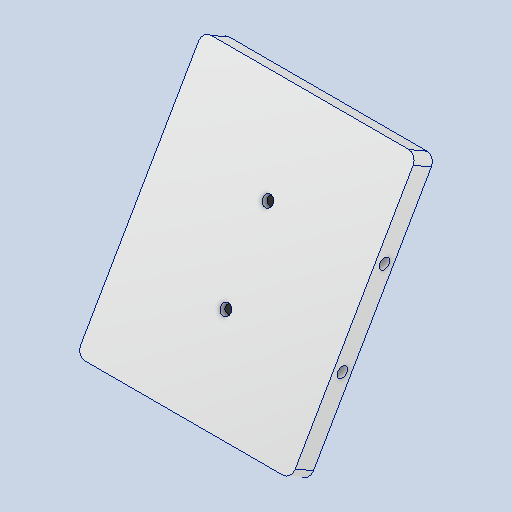
# Autodesk Inventor part: belt_liner_v5_Plate_3
Saved by Autodesk Inventor 2025.2 (Build 292293000, 293)
## iProperties
Created: 2025-02-23
Part Number: belt_liner_v5_Plate_3
Material: アルミニウム 6061
Document SubType Name: Modeling
Designer: haruy
Density: 2.7 g/cm^3
Appearance: アルミニウム - フラット
Author: haruy
Autodesk Inventor part; units mm, degrees
ref_plane "YZ Plane" through (0, 0, 0) normal (1, 0, 0) x (0, 1, 0)
ref_plane "XZ Plane" through (0, 0, 0) normal (0, 1, 0) x (-1, 0, 0)
ref_plane "XY Plane" through (0, 0, 0) normal (0, 0, 1) x (1, 0, 0)
derived "belt_liner_v5_Sketch_Base.ipt"
sketch "スケッチ1" plane through (300, 0, 0) normal (1, 0, 0) x (0, 1, 0)
  circle A0 centre (0, 0) radius 22.36 projected
  circle A1 centre (742.4003, -428.625) radius 23.875 construction
  line L0 (0, 0) -> (0, -985.832) projected
  line L1 (0, 0) -> (742.4003, -428.625) projected
  line L2 (-48.7433, -24.4258) -> (-56.2433, -37.4162) projected
  line L3 (-56.2433, -37.4162) -> (725.7777, -488.9162) projected
  line L4 (725.7777, -488.9162) -> (733.2777, -475.9258) projected
  line L5 (733.2777, -475.9258) -> (-48.7433, -24.4258) projected
  line L6 (-44.1225, 123.2584) -> (-44.1225, 123.2584) projected
  line L7 (0, -985.832) -> (0, 0) projected
  circle A2 centre (0, 0) radius 12.5 projected
  circle A3 centre (0, 0) radius 15 projected
  line L8 (0, 0) -> (0, 0) projected
  circle A4 centre (0, 0) radius 24.06 construction
  line L9 (0, 0) -> (0, 0) projected
  line L10 (0, 0) -> (0, 0) projected
  line L11 (-48.7433, -24.4258) -> (-46.2433, -20.0957) projected
  circle A5 centre (742.4003, -428.625) radius 5 projected
  line L12 (733.2777, -475.9258) -> (707.2969, -460.9258) projected
  line L13 (707.2969, -460.9258) -> (709.7969, -456.5957) projected
  line L14 (709.7969, -456.5957) -> (735.7777, -471.5957) projected
  line L15 (735.7777, -471.5957) -> (733.2777, -475.9258) projected
  circle A6 centre (738.0702, -426.125) radius 5.1 projected
  line L16 (742.4003, -428.625) -> (509.0943, -293.9257) projected
  circle A7 centre (759.7208, -438.625) radius 5.1 projected
  line L17 (740.6202, -421.7083) -> (762.2708, -434.2083) projected
  line L18 (735.5202, -430.5417) -> (757.1708, -443.0417) projected
  circle A8 centre (742.4003, -428.625) radius 22.175 construction
  circle A9 centre (738.0702, -426.125) radius 10.1 construction
  circle A10 centre (759.7208, -438.625) radius 10.1 construction
  line L19 (743.1202, -417.3781) -> (764.7708, -429.8781) construction
  line L20 (733.0202, -434.8719) -> (754.6708, -447.3719) construction
  line L21 (743.1202, -417.3781) -> (730.6598, -410.1842) construction
  line L22 (729.3233, -421.075) -> (734.3733, -412.3281) construction
  line L23 (764.7708, -429.8781) -> (770.9335, -433.4362) construction
  line L24 (770.9335, -433.4362) -> (771.2695, -433.6302) projected
  line L25 (754.6708, -447.3719) -> (764.7708, -429.8781) projected
  line L26 (764.7708, -429.8781) -> (773.431, -434.8781) projected
  line L27 (773.431, -434.8781) -> (763.331, -452.3719) projected
  line L28 (763.331, -452.3719) -> (754.6708, -447.3719) construction
  circle A11 centre (725.8674, -468.7607) radius 1.5 projected
  circle A12 centre (0, 0) radius 30 projected
  circle A13 centre (742.4003, -428.625) radius 6 construction
  circle A14 centre (0, 0) radius 24.06 construction
  circle A15 centre (0, 0) radius 24.06 projected
  circle A16 centre (742.4003, -428.625) radius 24.06 projected
  line L29 (754.4303, -407.7884) -> (12.03, 20.8366) projected
  circle A17 centre (725.8592, -419.075) radius 4 projected
  circle A18 centre (725.8592, -419.075) radius 1.5 projected
  circle A19 centre (742.4003, -428.625) radius 18.525 construction
  circle A20 centre (748.9869, -417.4167) radius 4 projected
  line L30 (737.4369, -437.4219) -> (742.4869, -428.675) projected
  circle A21 centre (748.9869, -417.4167) radius 1.5 projected
  line L31 (734.3733, -412.3281) -> (737.8233, -406.3526) construction
  line L32 (737.8233, -406.3526) -> (776.881, -428.9026) projected
  line L33 (773.431, -434.8781) -> (776.881, -428.9026) projected
  line L34 (737.8233, -406.3526) -> (723.6503, -415.7402) projected
  line L35 (720.8233, -435.7974) -> (759.881, -458.3474) projected
  line L36 (720.8233, -435.7974) -> (721.8667, -418.8295) projected
  line L37 (763.331, -452.3719) -> (759.881, -458.3474) projected
  circle A22 centre (735.9869, -439.9333) radius 4 projected
  circle A23 centre (735.9869, -439.9333) radius 1.5 projected
  circle A24 centre (717.2072, -463.7607) radius 1.5 projected
  circle A25 centre (742.4003, -428.625) radius 34.06 projected
  circle A26 centre (742.4869, -428.675) radius 8.5 projected
  line L38 (-57.9836, -13.421) -> (-72.9836, -13.421) projected
  line L39 (-72.9836, -13.421) -> (-72.9836, -278.421) projected
  line L40 (-72.9836, -278.421) -> (-57.9836, -278.421) projected
  line L41 (-57.9836, -278.421) -> (-57.9836, -13.421) projected
  line L42 (327.0164, -263.421) -> (-72.9836, -263.421) projected
  line L43 (-72.9836, -263.421) -> (-72.9836, -278.421) projected
  line L44 (-72.9836, -278.421) -> (327.0164, -278.421) projected
  line L45 (327.0164, -278.421) -> (327.0164, -263.421) projected
  line L46 (297.0164, -263.421) -> (297.0164, -278.421) projected
  line L47 (327.0164, -278.421) -> (361.1893, -278.421) projected
  line L48 (361.1893, -278.421) -> (368.6893, -265.4306) projected
  line L49 (-207.9836, 176.579) -> (-227.9836, 176.579) projected
  line L50 (-227.9836, 176.579) -> (-227.9836, -413.421) projected
  line L51 (-227.9836, -413.421) -> (-207.9836, -413.421) projected
  line L52 (-207.9836, -413.421) -> (-207.9836, 176.579) projected
  line L53 (-51.4069, -263.5692) -> (-53.919, -273.2486) projected
  line L54 (-53.919, -273.2486) -> (703.31, -469.7727) projected
  line L55 (703.31, -469.7727) -> (705.822, -460.0934) projected
  line L56 (705.822, -460.0934) -> (-51.4069, -263.5692) projected
  circle A27 centre (0, 0) radius 24.06 projected
  line L57 (1412.7204, 281.579) -> (-606.6364, 281.579) projected
  line L58 (1185.5776, -518.421) -> (-909.402, -518.421) projected
  line L59 (9.7721, 46.9258) -> (885.3238, -458.5742) projected
  line L60 (885.3238, -458.5742) -> (892.8238, -445.5838) projected
  line L61 (892.8238, -445.5838) -> (17.2721, 59.9162) projected
  line L62 (17.2721, 59.9162) -> (9.7721, 46.9258) projected
  line L63 (32.4276, 51.1662) -> (872.4722, -433.8338) projected
  line L64 (872.4722, -433.8338) -> (876.2222, -427.3386) projected
  line L65 (876.2222, -427.3386) -> (36.1776, 57.6614) projected
  line L66 (36.1776, 57.6614) -> (32.4276, 51.1662) projected
  line L67 (36.1776, 57.6614) -> (94.8941, 23.7614) projected
  line L68 (94.8941, 23.7614) -> (97.6441, 28.5245) projected
  line L69 (97.6441, 28.5245) -> (38.9276, 62.4245) projected
  line L70 (38.9276, 62.4245) -> (36.1776, 57.6614) projected
  circle A28 centre (218.0519, 108.5407) radius 120 projected
  line L71 (77.0164, 123.579) -> (57.0164, 123.579) projected
  line L72 (57.0164, 123.579) -> (57.0164, 103.579) projected
  line L73 (57.0164, 103.579) -> (77.0164, 103.579) projected
  line L74 (77.0164, 103.579) -> (77.0164, 123.579) projected
  line L75 (218.0519, 108.5407) -> (186.9936, 224.4518) projected
  line L76 (218.0519, 108.5407) -> (102.1408, 77.4824) projected
  line L77 (218.0519, 108.5407) -> (158.0519, 4.6177) projected
  line L78 (189.9936, 229.648) -> (99.1408, 72.2863) projected
  line L79 (99.1408, 72.2863) -> (93.9447, 75.2863) projected
  line L80 (93.9447, 75.2863) -> (184.7975, 232.648) projected
  line L81 (184.7975, 232.648) -> (189.9936, 229.648) projected
  line L82 (184.7975, 232.648) -> (181.7975, 227.4518) projected
  line L83 (181.7975, 227.4518) -> (177.4674, 229.9518) projected
  line L84 (177.4674, 229.9518) -> (180.4674, 235.148) projected
  line L85 (180.4674, 235.148) -> (184.7975, 232.648) projected
  line L86 (93.9447, 75.2863) -> (96.9447, 80.4824) projected
  line L87 (96.9447, 80.4824) -> (92.6146, 82.9824) projected
  line L88 (92.6146, 82.9824) -> (89.6146, 77.7863) projected
  line L89 (89.6146, 77.7863) -> (93.9447, 75.2863) projected
  line L90 (77.0164, 123.579) -> (117.0164, 123.579) projected
  line L91 (117.0164, 123.579) -> (117.0164, 103.579) projected
  line L92 (117.0164, 103.579) -> (77.0164, 103.579) projected
  line L93 (77.0164, 103.579) -> (77.0164, 123.579) projected
  circle A29 centre (218.0519, 108.5407) radius 132.0681 projected
  line L94 (103.6776, 174.5748) -> (38.9276, 62.4245) projected
  line L95 (32.4276, 51.1662) -> (11.6951, 15.2564) projected
  line L96 (11.6951, 15.2564) -> (20.3553, 10.2564) projected
  line L97 (20.3553, 10.2564) -> (41.0878, 46.1662) projected
  line L98 (41.0878, 46.1662) -> (32.4276, 51.1662) projected
  line L99 (152.0179, -5.8336) -> (158.0519, 4.6177) projected
  line L100 (152.0179, -5.8336) -> (20.3553, 10.2564) projected
  line L101 (74.8121, 3.6014) -> (78.3121, 9.6636) projected
  line L102 (78.3121, 9.6636) -> (92.5711, 1.4312) projected
  line L103 (181.7975, 227.4518) -> (154.2911, 210.1998) projected
  line L104 (96.9447, 80.4824) -> (98.1322, 112.9297) projected
  line L105 (99.1408, 72.2863) -> (116.3929, 44.7799) projected
  line L106 (-324.9836, 281.579) -> (-324.9836, -518.421) projected
  line L107 (1175.0164, 281.579) -> (1175.0164, -518.421) projected
  line L108 (17.2721, 59.9162) -> (9.7721, 46.9258) projected
  line L109 (9.7721, 46.9258) -> (-3.2183, 54.4258) projected
  line L110 (-3.2183, 54.4258) -> (4.2817, 67.4162) projected
  line L111 (4.2817, 67.4162) -> (17.2721, 59.9162) projected
  line L112 (-3.2183, 54.4258) -> (-5.7183, 50.0957) projected
  line L113 (-5.7183, 50.0957) -> (22.4276, 33.8457) projected
  line L114 (22.4276, 33.8457) -> (24.9276, 38.1758) projected
  line L115 (24.9276, 38.1758) -> (-3.2183, 54.4258) projected
  line L116 (-48.7433, -24.4258) -> (-46.2433, -20.0957) projected
  line L117 (-46.2433, -20.0957) -> (5.7183, -50.0957) projected
  line L118 (5.7183, -50.0957) -> (3.2183, -54.4258) projected
  line L119 (3.2183, -54.4258) -> (-48.7433, -24.4258) projected
  line L120 (789.6086, -403.313) -> (798.2689, -408.313) projected
  line L121 (798.2689, -408.313) -> (785.0364, -431.2324) projected
  line L122 (785.0364, -431.2324) -> (776.3761, -426.2324) projected
  line L123 (776.3761, -426.2324) -> (789.6086, -403.313) projected
  line L124 (885.3238, -458.5742) -> (882.8238, -462.9043) projected
  line L125 (882.8238, -462.9043) -> (856.843, -447.9043) projected
  line L126 (856.843, -447.9043) -> (859.343, -443.5742) projected
  line L127 (859.343, -443.5742) -> (885.3238, -458.5742) projected
  line L128 (7.6071, 48.1758) -> (11.9372, 45.6758) projected
  line L129 (11.9372, 45.6758) -> (19.4372, 58.6662) projected
  line L130 (19.4372, 58.6662) -> (15.1071, 61.1662) projected
  line L131 (15.1071, 61.1662) -> (7.6071, 48.1758) projected
  line L132 (19.4372, 58.6662) -> (14.4372, 50.0059) projected
  line L133 (14.4372, 50.0059) -> (24.8295, 44.0059) projected
  line L134 (24.8295, 44.0059) -> (29.8295, 52.6662) projected
  line L135 (29.8295, 52.6662) -> (19.4372, 58.6662) projected
  line L136 (931.2231, -485.0742) -> (935.5533, -487.5742) projected
  line L137 (935.5533, -487.5742) -> (951.5533, -459.8614) projected
  line L138 (951.5533, -459.8614) -> (947.2231, -457.3614) projected
  line L139 (947.2231, -457.3614) -> (931.2231, -485.0742) projected
  line L140 (944.4731, -462.1245) -> (934.9731, -478.579) projected
  line L141 (934.9731, -478.579) -> (919.3847, -469.579) projected
  line L142 (919.3847, -469.579) -> (928.8847, -453.1245) projected
  line L143 (928.8847, -453.1245) -> (944.4731, -462.1245) projected
  line L144 (924.1347, -461.3518) -> (939.7231, -470.3518) projected
  line L145 (926.6347, -457.0216) -> (921.6347, -465.6819) projected
  line L146 (921.6347, -465.6819) -> (882.6635, -443.1819) projected
  line L147 (882.6635, -443.1819) -> (887.6635, -434.5216) projected
  line L148 (887.6635, -434.5216) -> (926.6347, -457.0216) projected
  line L149 (888.9135, -432.3566) -> (881.4135, -445.347) projected
  line L150 (881.4135, -445.347) -> (874.4853, -441.347) projected
  line L151 (874.4853, -441.347) -> (881.9853, -428.3566) projected
  line L152 (881.9853, -428.3566) -> (888.9135, -432.3566) projected
  line L153 (31.0795, 54.8313) -> (23.5795, 41.8409) projected
  line L154 (23.5795, 41.8409) -> (30.5077, 37.8409) projected
  line L155 (30.5077, 37.8409) -> (38.0077, 50.8313) projected
  line L156 (38.0077, 50.8313) -> (31.0795, 54.8313) projected
  line L157 (16.9372, 54.3361) -> (27.3295, 48.3361) projected
  circle A30 centre (4.192, 47.2607) radius 1.25 projected
  circle A31 centre (12.8522, 42.2607) radius 1.25 projected
  line L158 (17.2721, 59.9162) -> (9.7721, 46.9258) projected
  line L159 (885.3238, -458.5742) -> (882.8238, -462.9043) projected
  line L160 (882.8238, -462.9043) -> (933.0533, -491.9043) projected
  line L161 (933.0533, -491.9043) -> (935.5533, -487.5742) projected
  line L162 (935.5533, -487.5742) -> (885.3238, -458.5742) projected
  line L163 (375.0164, 281.579) -> (375.0164, -518.421) projected
  line L164 (38.9276, 62.4245) -> (41.4276, 66.7546) projected
  line L165 (41.4276, 66.7546) -> (100.1441, 32.8546) projected
  line L166 (100.1441, 32.8546) -> (97.6441, 28.5245) projected
  line L167 (97.6441, 28.5245) -> (38.9276, 62.4245) projected
  line L168 (97.7242, 18.6633) -> (115.0447, 8.6633) projected
  line L169 (115.0447, 8.6633) -> (117.5447, 12.9934) projected
  line L170 (117.5447, 12.9934) -> (100.2242, 22.9934) projected
  line L171 (100.2242, 22.9934) -> (97.7242, 18.6633) projected
  line L172 (116.2947, 10.8284) -> (98.9742, 20.8284) projected
  line L173 (327.0164, -263.421) -> (335.2086, -263.421) projected
  line L174 (335.2086, -263.421) -> (342.7086, -250.4306) projected
  line L175 (-48.7433, -24.4258) -> (-56.2433, -37.4162) projected
  line L176 (-56.2433, -37.4162) -> (-77.8939, -24.9162) projected
  line L177 (-77.8939, -24.9162) -> (-70.3939, -11.9258) projected
  line L178 (-70.3939, -11.9258) -> (-48.7433, -24.4258) projected
  line L179 (-207.9836, -73.421) -> (-72.9836, -73.421) projected
  line L180 (-72.9836, -73.421) -> (-72.9836, -93.421) projected
  line L181 (-72.9836, -93.421) -> (-207.9836, -93.421) projected
  line L182 (-207.9836, -93.421) -> (-207.9836, -73.421) projected
  line L183 (-72.9836, -198.421) -> (-207.9836, -198.421) projected
  line L184 (-207.9836, -198.421) -> (-207.9836, -218.421) projected
  line L185 (-207.9836, -218.421) -> (-72.9836, -218.421) projected
  line L186 (-72.9836, -218.421) -> (-72.9836, -198.421) projected
  line L187 (-227.9836, -118.421) -> (-207.9836, -118.421) projected
  circle A32 centre (-30.1728, -32.2607) radius 1.25 projected
  circle A33 centre (-12.8522, -42.2607) radius 1.25 projected
  line L188 (-5.7183, 50.0957) -> (-46.2433, -20.0957) projected
  circle A34 centre (44.6769, 5.3827) radius 15 projected
  circle A35 centre (17.6769, -41.3827) radius 15 projected
  circle A36 centre (44.6769, 5.3827) radius 22 projected
  circle A37 centre (17.6769, -41.3827) radius 22 projected
  circle A38 centre (31.1769, -18) radius 3 projected
  line L189 (44.6769, 5.3827) -> (17.6769, -41.3827) projected
  circle A39 centre (26.7448, 25.5678) radius 3 projected
  circle A40 centre (-8.77, -35.9456) radius 3 projected
  circle A41 centre (866.7533, -450.7393) radius 1.25 projected
  circle A42 centre (875.4135, -455.7393) radius 1.25 projected
  circle A43 centre (994.8767, -339.9593) radius 120 projected
  line L190 (278.0519, 212.4638) -> (1054.8767, -236.0362) projected
  line L191 (-207.9836, -118.421) -> (1175.0164, -118.421) projected
  line L192 (-227.9836, -283.421) -> (-207.9836, -283.421) projected
  line L193 (-72.9836, -68.421) -> (-92.9836, -68.421) projected
  line L194 (-92.9836, -68.421) -> (-92.9836, -88.421) projected
  line L195 (-92.9836, -88.421) -> (-72.9836, -88.421) projected
  line L196 (-72.9836, -88.421) -> (-72.9836, -68.421) projected
  line L197 (-72.9836, -218.421) -> (-92.9836, -218.421) projected
  line L198 (-92.9836, -218.421) -> (-92.9836, -238.421) projected
  line L199 (-92.9836, -238.421) -> (-72.9836, -238.421) projected
  line L200 (-72.9836, -238.421) -> (-72.9836, -218.421) projected
  circle A44 centre (-28.7272, -34.6374) radius 15 projected
  line L201 (-92.9836, 143.579) -> (-112.9836, 143.579) projected
  line L202 (-112.9836, 143.579) -> (-112.9836, -340.421) projected
  line L203 (-112.9836, -340.421) -> (-92.9836, -340.421) projected
  line L204 (-92.9836, -340.421) -> (-92.9836, 143.579) projected
  line L205 (-98.6706, -321.2466) -> (-92.9836, -340.421) projected
  line L206 (-92.9836, -340.421) -> (762.3277, -86.7414) projected
  line L207 (762.3277, -86.7414) -> (756.6407, -67.567) projected
  line L208 (756.6407, -67.567) -> (-98.6706, -321.2466) projected
  line L209 (297.0164, -278.421) -> (282.0164, -278.421) projected
  line L210 (282.0164, -278.421) -> (282.0164, -293.421) projected
  line L211 (282.0164, -293.421) -> (297.0164, -293.421) projected
  line L212 (297.0164, -293.421) -> (297.0164, -278.421) projected
  line L213 (282.0164, -293.421) -> (267.0164, -293.421) projected
  line L214 (267.0164, -293.421) -> (267.0164, -210.9924) projected
  line L215 (267.0164, -210.9924) -> (282.0164, -210.9924) projected
  line L216 (282.0164, -210.9924) -> (282.0164, -293.421) projected
  line L217 (947.2231, -457.3614) -> (854.3308, -403.73) projected
  circle A45 centre (257.8891, 85.5407) radius 120 projected
  line L218 (-189.9836, 176.579) -> (-189.9836, -384.0126) projected
  point P0 (730.6598, -410.1842)
  point P1 (-65.4836, -23.421)
  point P2 (-65.4836, -270.921)
  point P3 (317.0164, -270.921)
  point P4 (307.0164, -270.921)
  point P5 (347.6105, -261.921)
  point P6 (356.2707, -266.921)
  point P7 (-42.9836, -270.921)
  point P8 (694.8867, -462.421)
  point P9 (57.0164, 113.579)
  point P10 (782.9924, -414.7727)
  point P11 (931.9289, -465.8518)
  point P12 (3.2183, -54.4258)
  point P13 (274.5164, -220.9924)
  constraints: 6 other
extrude "押し出し1" add sketch "スケッチ1" against normal blind 51 contours L117 A35 L118 L5 L0 | L0 L5 A37 L117 | A37 L5 A44 L117 | L117 L118 A35 | L117 A44 L5 L11 | L117 A44 L5 picked at (5.4712, -49.9824)
sketch "スケッチ3" plane through (249, 5.7183, -50.0957) normal (0, 0.5, 0.8660254) x (1, 0, 0)
  circle A0 centre (25.5, -40) radius 1.25
  line L0 (0, -60) -> (0, 0) projected
  line L1 (51, -60) -> (0, -60) projected
  circle A1 centre (25.5, -20) radius 1.25
  line L2 (51, 0) -> (51, -60) projected
  point P0 (-249, -30)
  dimension "d3" = 2.5
  dimension "d4" = 25.5
  dimension "d5" = 20
  dimension "d6" = 2.5
  dimension "d7" = 20
  dimension "d8" = 25.5
  constraints: 2 centre point
  measures "d3" diameter of A0
  measures "d4" distance from line of A0.centre L0
  measures "d5" distance from line of A0.centre L1
  measures "d6" diameter of A1
  measures "d7" distance of A0.centre A1.centre
  measures "d8" distance from line of L2 A1.centre
hole "穴1" at (274.5, -11.6022, -40.0957) at (274.5, -28.9228, -30.0957) direction (0, -0.5, -0.8660254) diameter 2.5 end through all
fillet "フィレット1" radius 2 4 edges at (300, -47.4933, -22.2607) (249, -47.4933, -22.2607) (300, 4.4683, -52.2607) (249, 4.4683, -52.2607)
equation "\"d7\" = d5"
equation "\"d8\" = d4"
